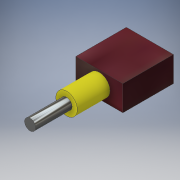
# Autodesk Inventor part: Switch
Saved by Autodesk Inventor 2016 (Build 200138000, 138)
## iProperties
Created: 2016-10-04
Part Number: Switch
Material: Generic
Document SubType Name: Modeling
Designer: desirw
Density: 1 g/cm^3
Appearance: Default
Author: desirw
Autodesk Inventor part; units mm, degrees
ref_plane "YZ Plane" through (0, 0, 0) normal (1, 0, 0) x (0, 1, 0)
ref_plane "XZ Plane" through (0, 0, 0) normal (0, 1, 0) x (-1, 0, 0)
ref_plane "XY Plane" through (0, 0, 0) normal (0, 0, 1) x (1, 0, 0)
sketch "Sketch1" plane through (0, 0, 0) normal (0, 0, 1) x (1, 0, 0)
  line L0 (2.1516, 4.7552) -> (14.9532, 4.7552)
  line L1 (14.9532, 4.7552) -> (14.9532, -2.1028)
  line L2 (14.9532, -2.1028) -> (2.1516, -2.1028)
  line L3 (2.1516, -2.1028) -> (2.1516, 4.7552)
  point P0 (0, 0)
  dimension "d0" = 12.8016
  dimension "d1" = 6.858
  constraints: 8 end point, 2 parallel, 1 horizontal, 1 perpendicular
  measures "d0" distance of L1.end L2.end
  measures "d1" distance of L0.end L1.end
extrude "Extrusion1" add sketch "Sketch1" along normal blind 13.7414
sketch "Sketch2" plane through (0, 0, 13.7414) normal (0, 0, 1) x (1, 0, 0)
  circle A0 centre (8.5524, 1.3262) radius 2.921
  line L0 (14.9532, -2.1028) -> (14.9532, 4.7552) projected
  line L1 (14.9532, 4.7552) -> (2.1516, 4.7552) projected
  point P0 (0, 0)
  dimension "d4" = 5.842
  dimension "d5" = 6.4008
  dimension "d6" = 3.429
  constraints: 1 centre point
  measures "d4" diameter of A0
  measures "d5" distance from line of L0 A0.centre
  measures "d6" distance from line of L1 A0.centre
extrude "Extrusion2" add sketch "Sketch2" along normal blind 8.89
sketch "Sketch3" plane through (8.5524, 1.3262, 22.6314) normal (0, 0, 1) x (1, 0, 0)
  circle A0 centre (0, 0) radius 1.4986
  point P0 (-8.5524, -1.3262)
  dimension "d9" = 2.9972
  constraints: 1 centre point
  measures "d9" diameter of A0
extrude "Extrusion3" add sketch "Sketch3" along normal blind 9.906
body "Solid1"
